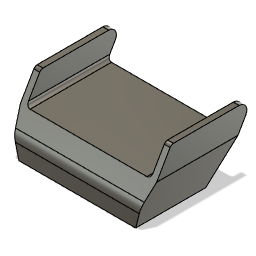
Fimi_Mount (Autodesk Fusion 360 design; units mm, degrees)
Autodesk Fusion 360 part; units mm, degrees
sketch "Skizze2" plane through (0, 0, 0) normal (1, 0, 0) x (0, 0, -1)
  line L0 (0, 0) -> (-36, 0)
  line L1 (0, 0) -> (11.547, 20)
  line L2 (11.547, 20) -> (-30.2265, 20)
  line L3 (-30.2265, 20) -> (-36, 10)
  line L4 (-36, 10) -> (-36, 0)
  dimension "d1" = 36
  dimension "d2" = 10
  dimension "d3" = 120
  dimension "d4" = 20
  constraint coincident L0.start L1.start
  constraint horizontal L0
  constraint parallel L0 L2
  constraint perpendicular L0 L4
  constraint parallel L1 L3
  measures "d1" distance of L0.start L0.end
  measures "d2" distance of L0.end L3.end
  measures "d3" angle of L0 L1
  measures "d4" distance of L0 L2
extrude "Extrusion1" add sketch "Skizze2" along normal mid plane 60
sketch "Skizze3" plane through (0, 0, 0) normal (0, -0.5, -0.866025) x (-1, 0, 0)
  line L0 (30, 23.094) -> (-30, 23.094)
  line L1 (-30, 23.094) -> (-30, 0)
  line L2 (-30, 0) -> (30, 0)
  line L3 (30, 0) -> (30, 23.094)
  line L4 (-30, 23.094) -> (-32, 23.094)
  line L5 (-32, 23.094) -> (-32, 28.021)
  line L6 (-32, 28.021) -> (-32, 38.094)
  line L7 (-32, 38.094) -> (-35, 38.094)
  line L8 (-35, 38.094) -> (-35, 23.094)
  line L9 (-35, 23.094) -> (-30, 0)
  line L10 (-30, 0) -> (-30, 23.094)
  line L11 (0, 0) -> (0, 23.094) construction
  line L12 (35, 38.094) -> (35, 23.094)
  line L13 (32, 23.094) -> (32, 28.021)
  line L14 (30, 23.094) -> (30, 0)
  line L15 (30, 23.094) -> (32, 23.094)
  line L16 (35, 23.094) -> (30, 0)
  line L17 (32, 28.021) -> (32, 38.094)
  line L18 (32, 38.094) -> (35, 38.094)
  line L19 (30, 0) -> (30, 23.094)
  dimension "d7" = 2
  dimension "d9" = 3
  dimension "d10" = 15
  constraint coincident L0.end L1.start
  constraint perpendicular L1 L4
  constraint perpendicular L4 L5
  constraint perpendicular L4 L6
  constraint perpendicular L6 L7
  constraint perpendicular L7 L8
  constraint coincident L1.end L2.start
  constraint coincident L4 L8.end
  constraint coincident L11.start origin
  constraint midpoint L0 L11.end
  constraint symmetric L0.end L11 L0.start
  constraint symmetric L1.end L11 L2.end
  constraint symmetric L4.end L11 L13.start
  constraint symmetric L5.end L11 L13.end
  constraint symmetric L6.end L11 L17.end
  constraint symmetric L7.end L11 L12.start
  constraint symmetric L8.end L11 L12.end
  measures "d7" distance of L0.end L4.end
  measures "d9" distance of L6.end L7.end
  measures "d10" distance of L4 L7
sweep "Sweeping1" add profiles "Skizze3" along 1 edges at (-30, 20, 9.3397) section 1 contours L3 L12 L13 L14 L15 L16 L17 L18 L19 | L1 L4 L5 L6 L7 L8 L9 L10
fillet "Abrundung1" radius 2 2 edges at (-32, 20, 9.3397) (32, 20, 9.3397)
sketch "Skizze4" plane through (-30, 0, 0) normal (1, 0, 0) x (0, 0, -1)
  line L0 (-36, 0) -> (-36, 10)
  line L1 (-36, 10) -> (-41.7735, 0)
  line L2 (-41.7735, 0) -> (-36, 0)
extrude "Extrusion2" cut sketch "Skizze4" against normal blind 4
extrude "Extrusion3" cut 1 faces at (30, 3.3333, 37.9245) along direction (1, 0, 0) blind 8
fillet "Abrundung2" radius 4 2 edges at (33.5, 32.9904, -19.047) (-33.5, 32.9904, -19.047)
fillet "Abrundung3" radius 2 2 edges at (-33.5, 32.9904, 22.7265) (33.5, 32.9904, 22.7265)
fillet "Abrundung4" radius 10 1 edges at (0, 10, 36)
